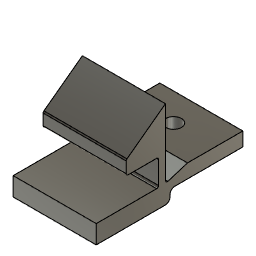
Base Plate Latch (Autodesk Fusion 360 design; units mm, degrees)
Autodesk Fusion 360 part; units mm, degrees
sketch "Sketch1" plane through (0, 0, 0) normal (1, 0, 0) x (0, 1, 0)
  line L0 (0, 0) -> (0, 4)
  line L1 (0, 4) -> (15, 4)
  line L2 (15, 4) -> (19.7697, 5.5)
  line L3 (19.7697, 5.5) -> (31.7697, 5.5)
  line L4 (31.7697, 5.5) -> (31.7697, 2.5)
  line L5 (31.7697, 2.5) -> (16, 2.5)
  line L6 (16, 2.5) -> (16, 0)
  line L7 (16, 0) -> (0, 0)
  dimension "d1" = 16
  dimension "d2" = 2.5
  dimension "d3" = 15
  dimension "d4" = 5
  dimension "d5" = 4
  dimension "d6" = 12
  dimension "d7" = 3
  constraint coincident L0.start L7.end
  constraint vertical L0
  constraint perpendicular L0 L1
  constraint perpendicular L0 L3
  constraint perpendicular L3 L4
  constraint perpendicular L0 L5
  constraint perpendicular L5 L6
  constraint perpendicular L0 L7
  measures "d1" distance of L6.end L0.start
  measures "d2" distance of L5.end L6.end
  measures "d3" distance of L0.end L1.end
  measures "d4" distance of L1.end L2.end
  measures "d5" distance of L0.start L0.end
  measures "d6" distance of L2.end L3.end
  measures "d7" distance of L3.end L4.end
extrude "Extrude1" add sketch "Sketch1" along normal blind 18
sketch "Magnet Slot" plane through (18, 0, 0) normal (1, 0, 0) x (0, 1, 0)
  line L0 (16, 0) -> (16, 2.5)
  line L1 (16, 2.5) -> (31.7697, 2.5)
  line L2 (31.7697, 2.5) -> (31.7697, 5.5)
  line L3 (31.7697, 5.5) -> (19.7697, 5.5)
  line L4 (19.7697, 5.5) -> (15, 4)
  line L5 (15, 4) -> (0, 4)
  line L6 (0, 4) -> (0, 0)
  line L7 (0, 0) -> (16, 0)
  line L8 (0, 0) -> (15, 0) construction
  line L9 (15, 0) -> (15, 4) construction
  line L10 (15, 4) -> (0, 4) construction
  line L11 (0, 4) -> (0, 0) construction
  line L12 (0.6, 0.6) -> (14.4, 0.6)
  line L13 (14.4, 0.6) -> (14.4, 3.4)
  line L14 (14.4, 3.4) -> (0.6, 3.4)
  line L15 (0.6, 3.4) -> (0.6, 0.6)
  dimension "d11" = -0.6
  constraint horizontal L8
  constraint vertical L9
  constraint horizontal L10
  constraint vertical L11
  constraint coincident L4.end L5.start
  constraint coincident L6.end L7.start
sketch "Sketch4" plane through (0, 0, 4) normal (0, 0, 1) x (-1, 0, 0)
  line L0 (0, -15) -> (0, 0)
  line L1 (0, 0) -> (-18, 0)
  line L2 (-18, 0) -> (-18, -15)
  line L3 (-18, -15) -> (0, -15)
  circle A0 centre (-9, -6) radius 3.5
  line L4 (-9, -9.5) -> (0, -9.5) construction
  dimension "d14" = 7
  constraint coincident A0 L4.start
  constraint coincident L0 L4.end
  constraint tangent A0 L4
  constraint perpendicular L0 L4
  measures "d14" diameter of A0
fillet "Fillet2" radius 1 2 edges at (9, 16, 2.5) (9, 16, 0)
sketch "Sketch6" plane through (0, 0, 0) normal (-1, 0, 0) x (0, -1, 0)
  arc A0 (-16, 1) -> (-15, 0) centre (-15, 1) ccw
  line L0 (-15, 0) -> (0, 0)
  line L1 (0, 0) -> (0, 4)
  line L2 (0, 4) -> (-15, 4)
  line L3 (-15, 4) -> (-19.7697, 5.5)
  line L4 (-19.7697, 5.5) -> (-31.7697, 5.5)
  line L5 (-31.7697, 5.5) -> (-31.7697, 2.5)
  line L6 (-31.7697, 2.5) -> (-17, 2.5)
  arc A1 (-16, 1.5) -> (-17, 2.5) centre (-17, 1.5) ccw
  line L7 (-16, 1.5) -> (-16, 1)
  line L8 (-9.5, 4) -> (-9.5, 0) construction
  line L9 (-13.5, 4) -> (-13.5, 9.7)
  line L10 (-13.5, 9.7) -> (-6.5, 9.7)
  line L11 (-6.5, 9.7) -> (-6.5, 12.7)
  line L12 (-15, 19) -> (-15, 4)
  line L13 (-6.5, 12.7) -> (-15, 19)
  point P0 (-9.5, 4)
  dimension "d37" = 1.5
  dimension "d38" = 4
  dimension "d39" = 5.7
  dimension "d41" = 7
  dimension "d42" = 15
  dimension "d48" = 3
  constraint coincident L2 P0
  constraint coincident L0 L8.end
  constraint perpendicular L0 L8
  constraint coincident L2 L9.start
  constraint perpendicular L2 L9
  constraint perpendicular L9 L10
  constraint perpendicular L10 L11
  constraint coincident L2 L3.start
  constraint perpendicular L2 L12
  measures "d37" distance of L9 L12
  measures "d38" distance of L9 P0
  measures "d39" distance of L9.start L9.end
  measures "d41" distance of L9.end L10.end
  measures "d42" distance of L12.start L2.end
  measures "d48" distance of L10.end L11.end
extrude "Extrude4" add sketch "Sketch6" against normal up to surface (18 mm away) contours L2 L9 L10 L11 L12 L13
sketch "Sketch5" plane through (0, 0, 5.5) normal (0, 0, 1) x (-1, 0, 0)
  line L0 (0, -31.7697) -> (0, -19.7697)
  line L1 (0, -19.7697) -> (-18, -19.7697)
  line L2 (-18, -19.7697) -> (-18, -31.7697)
  line L3 (-18, -31.7697) -> (0, -31.7697)
  line L4 (-18, -31.7697) -> (0, -19.7697) construction
  line L5 (0, -31.7697) -> (-18, -19.7697) construction
  circle A0 centre (-9, -25.7697) radius 2 construction
  dimension "d24" = 4
  constraint coincident L2.end L3.start
  constraint coincident L0.end L1.start
  constraint coincident L0.start L3.end
  constraint coincident L1.end L2.start
  constraint midpoint L5 A0.centre
  measures "d24" diameter of A0
hole "Hole3" at (9, 25.7697, 5.5) direction (0, 0, -1) diameter 3.4 depth 4 tip angle 118
fillet "Fillet4" radius 0.4 5 edges at (9, 13.5, 4) (9, 15, 4) (9, 13.5, 9.7) (9, 6.5, 9.7) (9, 6.5, 12.7)
